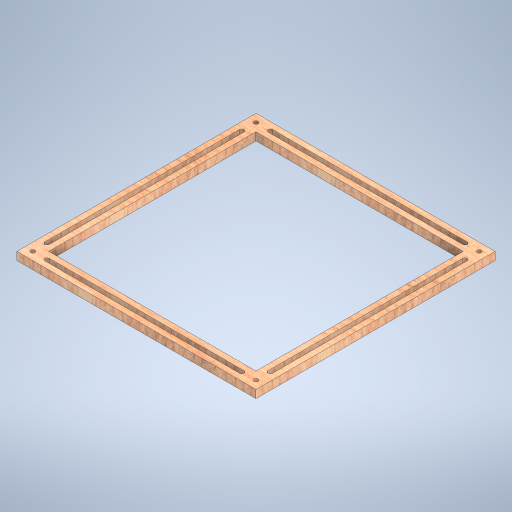
# Autodesk Inventor part: XYbase
Saved by Autodesk Inventor 2023 (Build 270158000, 158)
## iProperties
Created: 2023-10-26
Part Number: XYbase
Material: Wood (Birch)
Document SubType Name: Modeling
Designer: Mustapha
Density: 0.55 g/cm^3
Appearance: Birch - Natural Polished
Mass: 76.6201 g
Surface Area: 632.042 cm^2
Volume: 139.309 cm^3
Author: Mustapha
Autodesk Inventor part; units mm, degrees
ref_plane "YZ Plane" through (0, 0, 0) normal (1, 0, 0) x (0, 1, 0)
ref_plane "XZ Plane" through (0, 0, 0) normal (0, 1, 0) x (-1, 0, 0)
ref_plane "XY Plane" through (0, 0, 0) normal (0, 0, 1) x (1, 0, 0)
sketch "Sketch1" plane through (0, 0, 0) normal (0, 1, 0) x (-1, 0, 0)
  line L0 (0, 0) -> (300, 0)
  line L1 (300, 0) -> (300, -300)
  line L2 (300, -300) -> (0, -300)
  line L3 (0, -300) -> (0, 0)
  line L4 (20, -20) -> (280, -20)
  line L5 (280, -20) -> (280, -280)
  line L6 (280, -280) -> (20, -280)
  line L7 (20, -280) -> (20, -20)
  line L8 (150, 0) -> (150, -333.0511)
  line L9 (300, -150) -> (0, -150)
  line L10 (290, -23.4629) -> (290, -392.3608)
  line L11 (268.156, -10) -> (-9.9722, -10)
  line L12 (290, -27.75) -> (290, -272.25) construction
  line L13 (292.75, -27.75) -> (292.75, -272.25)
  line L14 (287.25, -272.25) -> (287.25, -27.75)
  arc A0 (292.75, -27.75) -> (287.25, -27.75) centre (290, -27.75) ccw
  arc A1 (287.25, -272.25) -> (292.75, -272.25) centre (290, -272.25) ccw
  line L15 (7.25, -27.75) -> (7.25, -272.25)
  line L16 (12.75, -272.25) -> (12.75, -27.75)
  arc A2 (12.75, -27.75) -> (7.25, -27.75) centre (10, -27.75) ccw
  arc A3 (7.25, -272.25) -> (12.75, -272.25) centre (10, -272.25) ccw
  line L17 (27.75, -10) -> (272.25, -10) construction
  line L18 (27.75, -12.75) -> (272.25, -12.75)
  line L19 (272.25, -7.25) -> (27.75, -7.25)
  arc A4 (27.75, -7.25) -> (27.75, -12.75) centre (27.75, -10) ccw
  arc A5 (272.25, -12.75) -> (272.25, -7.25) centre (272.25, -10) ccw
  line L20 (27.75, -287.25) -> (272.25, -287.25)
  line L21 (272.25, -292.75) -> (27.75, -292.75)
  arc A6 (27.75, -287.25) -> (27.75, -292.75) centre (27.75, -290) ccw
  arc A7 (272.25, -292.75) -> (272.25, -287.25) centre (272.25, -290) ccw
  line L22 (280, -280) -> (300, -300)
  circle A8 centre (290, -290) radius 2.75
  circle A9 centre (10, -290) radius 2.75
  circle A10 centre (290, -10) radius 2.75
  circle A11 centre (10, -10) radius 2.75
  point P0 (150, -20)
  point P1 (290, -150)
  point P2 (290, -25)
  point P3 (290, -275)
  point P4 (150, -10)
  point P5 (25, -10)
  point P6 (275, -10)
  point P7 (275, -290)
  dimension "d0" = 300
  dimension "d1" = 300
  dimension "d2" = 20
  dimension "d3" = 20
  dimension "d4" = 20
  dimension "d5" = 20
  dimension "d6" = 20
  dimension "d7" = 20
  dimension "d8" = 5.5
  dimension "d9" = 250
  dimension "d10" = 5.5
  dimension "d11" = 250
  dimension "d12" = 5.5
  dimension "d15" = 280
  constraints: 50 end point, 20 point on circle, 16 symmetric about line, 12 centre point, 8 tangent, 7 midpoint, 6 parallel, 6 point on line, 3 perpendicular, 2 horizontal, 2 vertical, 7 other
  measures "d0" distance between parallel lines of L3 L1
  measures "d1" distance between parallel lines of L2 L0
  measures "d2" distance of L8.start point (150, -20)
  measures "d3" distance between parallel lines of L2 L6
  measures "d4" distance between parallel lines of L5 L1
  measures "d5" distance between parallel lines of L3 L7
  measures "d6" diameter of L1 L10
  measures "d7" diameter of L0 L11
  measures "d8" distance between parallel lines of L14 L13
  measures "d9" distance of point (290, -25) point (290, -275)
  measures "d10" distance between parallel lines of L18 L19
  measures "d11" distance of point (25, -10) point (275, -10)
  measures "d12" diameter of A8
  measures "d15" diameter of L17 L9
extrude "Extrusion1" add sketch "Sketch1" along normal blind 10 contours L0 L8 L19 A4 L11 A11 L3 | L0 L1 L9 L13 A0 L14 L5 L4 L8 L18 A5 L19 | L11 A11 A4 L18 L8 L4 L7 L9 L16 A2 L15 L3 | L9 L15 A3 L16 L7 L6 L8 L20 A6 L21 L2 L3 | L1 L22 A8 L10 A1 L13 L9 | L2 L10 A8 L22 | L8 L21 A7 L20 L6 L22 A8 L10 L2 | L14 A1 L10 A8 L22 L5 L9
body "Solid1"
